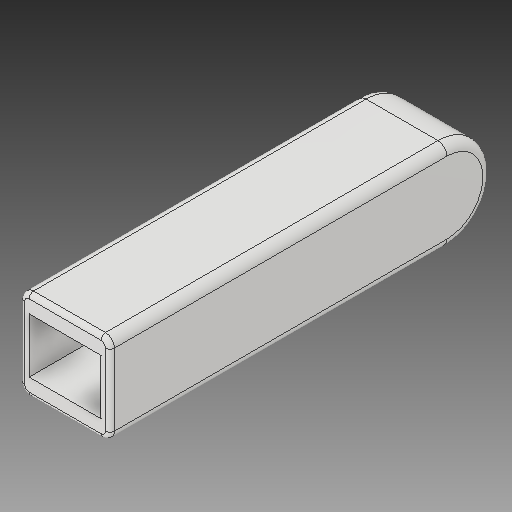
# Autodesk Inventor part: Part5_GOMA
Saved by Autodesk Inventor 2019 (Build 230136000, 136)
## iProperties
Created: 2018-10-25
Part Number: Part5_GOMA
Material: Polystyrene
Document SubType Name: Modeling
Designer: Isaac
Density: 1.021 g/cm^3
Appearance: Smooth - White
Mass: 17.6033 g
Surface Area: 114.508 cm^2
Volume: 17.2412 cm^3
Author: Isaac
Autodesk Inventor part; units mm, degrees
ref_plane "YZ Plane" through (0, 0, 0) normal (1, 0, 0) x (0, 1, 0)
ref_plane "XZ Plane" through (0, 0, 0) normal (0, 1, 0) x (-1, 0, 0)
ref_plane "XY Plane" through (0, 0, 0) normal (0, 0, 1) x (1, 0, 0)
sketch "Sketch1" plane through (0, 0, 0) normal (1, 0, 0) x (0, 1, 0)
  line L0 (10, 37.5) -> (10, -37.5)
  arc A0 (-10, -37.5) -> (10, -37.5) centre (0, -37.5) ccw
  line L1 (-10, -37.5) -> (-10, 37.5)
  line L2 (-10, 37.5) -> (10, 37.5)
  point P0 (0, 0)
  point P1 (-10, 0)
  dimension "d0" = 20
  dimension "d1" = 75
  dimension "d2" = 10
  constraints: 6 end point, 2 point on circle, 2 tangent, 1 centre point, 1 horizontal alignment, 1 midpoint, 1 parallel, 1 perpendicular, 1 vertical, 1 vertical alignment
  measures "d0" distance of L1.end L0.start
  measures "d1" distance of L0.start L0.end
  measures "d2" radius of A0
extrude "Extrusion1" add sketch "Sketch1" along normal mid plane 20
sketch "Sketch2" plane through (0, 0, 0) normal (1, 0, 0) x (0, 1, 0)
  line L0 (-10, 37.5) -> (10, 37.5) projected
  line L1 (6.1, 37.5) -> (6.1, -37.5)
  arc A0 (-6.1, -37.5) -> (6.1, -37.5) centre (0, -37.5) ccw
  line L2 (-6.1, -37.5) -> (-6.1, 37.5)
  point P0 (0, 0)
  dimension "d5" = 75
  dimension "d6" = 12.2
  constraints: 4 end point, 2 point on circle, 2 point on line, 2 tangent, 1 centre point, 1 perpendicular, 1 vertical, 1 vertical alignment
  measures "d5" distance of L1.start L1.end
  measures "d6" distance between parallel lines of L2 L1
extrude "Extrusion2" cut sketch "Sketch2" along normal mid plane 16
fillet "Fillet1" radius 2 6 edges at (-10, 0, -47.5) (-10, 10, 0) (-10, -10, 0) (10, 0, -47.5) (10, 10, 0) (10, -10, 0)
fillet "Fillet2" radius 1 8 edges at (-9.4142, -9.4142, 37.5) (-10, 0, 37.5) (-9.4142, 9.4142, 37.5) (0, 10, 37.5) (9.4142, 9.4142, 37.5) (10, 0, 37.5) (9.4142, -9.4142, 37.5) (0, -10, 37.5)
body "Solid1"
